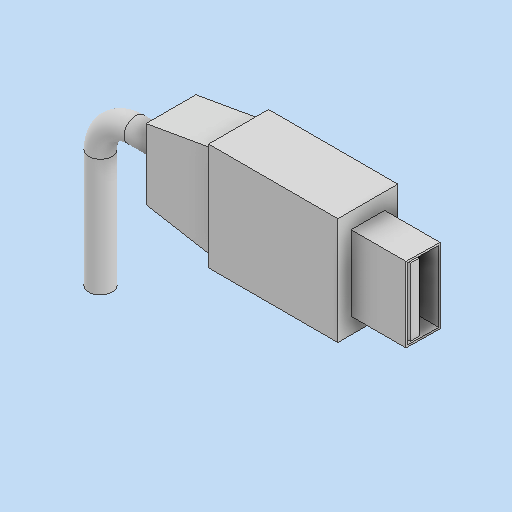
# Autodesk Inventor part: P00173-09-013
Saved by Autodesk Inventor 2022 (Build 260153070, 153G)
## iProperties
Created: 2021-07-09
Part Number: P00173-09-013
Material: Generic
Document SubType Name: Modeling
Designer: MPM
Density: 1 g/cm^3
Appearance: Default
Description: USB CABLE
Author: MPM
Comments: M2-Paypad 3d files for a Cardano blockchain payment terminal. Copyright (C) 2021 Maarten Menheere This program is free software; you can redistribute it and/or modify it under the terms of the GNU General Public License as published by the Free Software Foundation; either version 2 of the License, or (at your option) any later version. This program is distributed in the hope that it will be useful, but WITHOUT ANY WARRANTY; without even the implied warranty of MERCHANTABILITY or FITNESS FOR A PARTICULAR PURPOSE.  See the GNU General Public License for more details. You should have received a copy of the GNU General Public License along with this program; if not, write to the Free Software Foundation, Inc., 51 Franklin Street, Fifth Floor, Boston, MA  02110-1301, USA.
Autodesk Inventor part; units mm, degrees
derived "P00173-09-002.ipt"
sketch "USB_Position" plane through (50, 0, 12.5) normal (0, 0, 1) x (1, 0, 0)
  line L0 (-12.075, -35.5) -> (20.925, -35.5)
  line L1 (20.925, -35.5) -> (20.925, -32)
  line L2 (20.925, -32) -> (-12.075, -32)
  line L3 (-12.075, -32) -> (-12.075, -35.5)
  line L4 (-12.075, -13.5) -> (20.925, -13.5)
  line L5 (20.925, -13.5) -> (20.925, -10)
  line L6 (20.925, -10) -> (-12.075, -10)
  line L7 (-12.075, -10) -> (-12.075, -13.5)
  line L8 (22.425, -27) -> (-12.075, -27)
  line L9 (-12.075, -27) -> (-12.075, -18.5)
  line L10 (22.425, -18.5) -> (22.425, -27)
  line L11 (-12.075, -18.5) -> (22.425, -18.5)
  line L12 (21.925, -22.75) -> (22.425, -22.75)
  line L13 (21.925, -22.75) -> (21.925, 0) construction
  point P0 (-50, 0)
  point P1 (0.9654, 0)
sketch "USB_Side" plane through (72.425, -22.75, 12.5) normal (0, 1, 0) x (-1, 0, 0)
  line L0 (29.0554, 10.7) -> (7.0554, 10.7)
  line L1 (7.0554, 10.7) -> (7.0554, 0.5)
  line L2 (7.0554, 0.5) -> (29.0554, 0.5)
  line L3 (29.0554, 0.5) -> (29.0554, 10.7)
  line L4 (40.5554, 9.85) -> (29.0554, 9.85)
  line L5 (29.0554, 9.85) -> (29.0554, 1.35)
  line L6 (29.0554, 1.35) -> (40.5554, 1.35)
  line L7 (40.5554, 1.35) -> (40.5554, 9.85)
  line L8 (7.0554, 8.45) -> (-2.5446, 8.45)
  line L9 (-2.5446, 8.45) -> (-2.5446, 2.75)
  line L10 (-2.5446, 2.75) -> (7.0554, 2.75)
  line L11 (7.0554, 2.75) -> (7.0554, 8.45)
  line L12 (-2.5446, 9.1) -> (-2.9446, 9.1)
  line L13 (-2.9446, 9.1) -> (-2.9446, 2.1)
  line L14 (-2.9446, 2.1) -> (-2.5446, 2.1)
  line L15 (-2.5446, 2.1) -> (-2.5446, 9.1)
  line L16 (-2.5446, 5.6) -> (40.5554, 5.6) construction
  line L17 (-2.5896, -9.1065) -> (-2.2446, 10.6562)
  point P0 (72.425, -12.5)
  point P1 (29.0554, 5.6)
  point P2 (7.0554, 5.6)
  point P3 (-2.9446, 5.6)
  point P4 (34, 0)
  point P5 (34.5, 0)
  point P6 (34, 0)
  point P7 (-2.2831, 8.45)
  point P8 (-2.3826, 2.75)
  point P9 (7.0554, 2.75)
  point P10 (29.0554, 9.85)
ref_plane "Work Plane1" through (31.8696, -22.75, 18.1) normal (0, 0, 1) x (1, 0, 0)
sketch "Sketch3" plane through (31.8696, -22.75, 18.1) normal (0, 0, 1) x (1, 0, 0)
  line L0 (0, 0) -> (-6, 0)
  line L1 (43.1, 0) -> (0, 0) construction
  arc A0 (-6, 0) -> (-12, -6) centre (-6, -6) ccw
  line L2 (-12, -6) -> (-12, -26)
  point P0 (-31.8696, 22.75)
  dimension "d7" = 6
  dimension "d8" = 6
  dimension "d9" = 20
  constraints: 4 end point, 2 point on circle, 2 tangent, 1 centre point, 1 collinear, 1 perpendicular
  measures "d7" distance of L0.start L0.end
  measures "d8" radius of A0
  measures "d9" distance of L2.start L2.end
ref_plane "Work Plane2" through (31.8696, -22.75, 18.1) normal (-1, 0, 0) x (0, -1, 0)
ref_plane "Work Plane3" through (74.9696, -22.75, 18.1) normal (-1, 0, 0) x (0, -1, 0)
sketch "Sketch5" plane through (74.9696, -22.75, 18.1) normal (-1, 0, 0) x (0, -1, 0)
  line L0 (6.25, 2.85) -> (-6.25, 2.85)
  line L1 (-6.25, 2.85) -> (-6.25, -2.85)
  line L2 (-6.25, -2.85) -> (6.25, -2.85)
  line L3 (6.25, -2.85) -> (6.25, 2.85)
  line L4 (5.75, 2.15) -> (-5.75, 2.15)
  line L5 (-5.75, 2.15) -> (-5.75, 0.65)
  line L6 (-5.75, 0.65) -> (5.75, 0.65)
  line L7 (5.75, 0.65) -> (5.75, 2.15)
  line L8 (0, 2.15) -> (0, 2.85) construction
  line L9 (-6.05, 2.65) -> (6.05, 2.65)
  line L10 (6.05, 2.65) -> (6.05, -2.65)
  line L11 (6.05, -2.65) -> (-6.05, -2.65)
  line L12 (-6.05, -2.65) -> (-6.05, 2.65)
  point P0 (-22.75, -18.1)
  point P1 (0, -2.85)
  point P2 (0, -2.85)
  point P3 (0, -2.85)
  point P4 (0, -2.85)
  dimension "d14" = 0.7
  dimension "d15" = 0.5
  dimension "d16" = 0.2
  dimension "d17" = 1.5
  dimension "d18" = 12.5
  constraints: 26 end point, 7 perpendicular, 3 midpoint, 2 coincident, 1 horizontal, 3 other
  measures "d14" distance between parallel lines of L0 L4
  measures "d15" distance between parallel lines of L3 L7
  measures "d16" distance between parallel lines of L0 L9
  measures "d17" distance of L4.end L5.end
  measures "d18" distance of L1.end L2.end
sketch "Sketch4" plane through (31.8696, -22.75, 18.1) normal (-1, 0, 0) x (0, -1, 0)
  circle A0 centre (0, 0) radius 2
  point P0 (-22.75, -18.1)
  dimension "d10" = 4
  constraints: 1 centre point, 1 coincident
  measures "d10" diameter of A0
sweep "Sweep1" add profiles "Sketch4" path "Sketch3"
extrude "Extrusion1" add sketch "USB_Side" along normal mid plane 18.25 separate body contours L3 L2 L1 L0
extrude "Extrusion2" add sketch "USB_Side" along normal mid plane 12.75 contours L1 L10 L17 L8 bodies 2
extrude "Extrusion3" add sketch "USB_Side" along normal mid plane 16 contours L4 L7 L6 L3 bodies 2
draft "FaceDraft1" angle 10 pull direction (-1, 0, 0) faces at (35.7029, -14.75, 16.6833) (35.7029, -30.75, 16.6833) fixed edges at (43.3696, -14.75, 18.1) (43.3696, -30.75, 18.1)
extrude "Extrusion4" cut sketch "Sketch5" along normal blind 7.5 contours L9 L10 L11 L12 bodies 2
body "Solid1"
body "Solid2"
